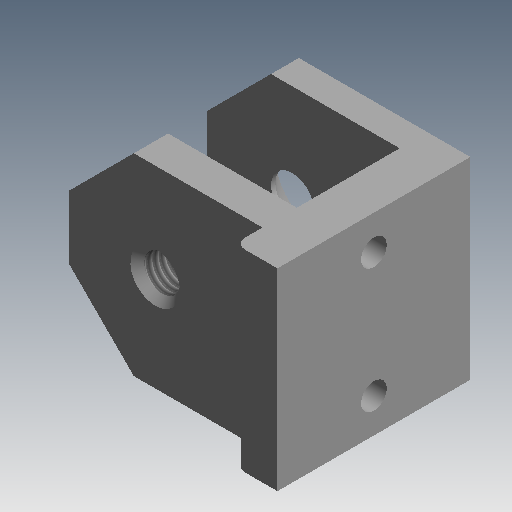
# Autodesk Inventor part: HBLTBBN45-SET_b
Saved by Autodesk Inventor 2020 (Build 240168000, 168)
## iProperties
Part Number: HBLTBBN45-SET_b
Material: 一般
Catalog Web Link: www.cadenas.de
Description: HBLTBA, HBLTBBNb-Free Angle Brackets - 20, 30, 40, 45 Square
Vendor: MISUMI
Document SubType Name: Modeling
Designer: partserver
Manufacturer: MISUMI
Mass: 44.0756 g
Surface Area: 143.656 cm^2
Volume: 44.0756 cm^3
Density: 1 g/cm^3
Appearance: PSOLRGB-192-192-192
Category: PARTsolutions
Company: MISUMI
PSOL_IDENT_0: {$CADENAS_DATA\23d-libs\misumi\metric\38_al_extrusions_blackets\hbltba.prj},183 {VTYP=3D},{NB=HBLTBB
PSOL_IDENT_1: N45-SET_b},{LINA=HBLTBBN45-SET},{NN=HBLTBA, HBLTBBNb},{DATE=08.06.2021 08:27:27},{GEOMDATE=18.10.201
PSOL_IDENT_2: 8 04:54:00},{VERSION=},{LINEID=100},{WBVAR=ALT1},{WBNUMERIC=}  {NB=HBLTBBN45-SET_b},{LINA=HBLTBBN45-
PSOL_IDENT_3: SET},{KT=DUMMY},{PN=HBLTBBN45-SET},{TP=HBLTBBN},{NO=45},{TNS=HBLTBBN45},{MATMB=A6N01SS-T5(Aluminum)(
PSOL_IDENT_4: EN AC-51400_AlMgSiO,7-T5)},{MATAB=SCM435(4137 Alloy Steel)(1.7220_34CrMo4)},{STMB=Alumite},{STAB=Tri
PSOL_IDENT_5: valent Chromate},{CS=45 Square (HFS8-45)},{A=45},{MA=6},{MAN=6},{N=-},{NN=0.0},{T=10},{TT1=6.5},{TT2=
PSOL_IDENT_6: 8.0},{W=24.0},{H=35},{H1=55},{E=29},{EN=29.0},{F=8},{FN=8.0},{C=15},{CN=15},{M=10},{L=16},{MASS=116.
PSOL_IDENT_7: 0},{AHS=M10x16},{ALT1=-SET},{ALT1ATT= '' , 'w/o Applicable Bolt and Nut Set' , '-SET' , 'with SET (A
PSOL_IDENT_8: pplicable Bolt and Nut Set)'   },{UM=-},{ACB=CBM6-35},{ACBD=6},{ACBDM=6},{ACBNO=6},{ACBL=35},{ACBQ=2
PSOL_IDENT_9: },{ACN=HDJFSN8-45},{ACNO=8-45},{ACNQ=1},{MATN=1010 Steel (or Equivalent)},{X=4},{MD=11.0},{AS=20.0},
PSOL_IDENT_10: {ES=5.5},{HFSH=6.000},{CPBL=27.6}
NB: HBLTBBN45-SET_b
NN: HBLTBA, HBLTBBNb
NT: Free Angle Brackets - 20, 30, 40, 45 Square
NBSYN: $PN._b
LINA: HBLTBBN45-SET
CATALOG: Misumi
PN: HBLTBBN45-SET
TNS: HBLTBBN45
MATMB: A6N01SS-T5
MATAB: 4137 Alloy Steel
STMB: Clear Anodizing
STAB: Trivalent Chromate Plating
CS: 45 Square (HFS8-45)
A: 45
MA: 6
N: -
T: 10
TT1: 6.5
TT2: 8
W: 24
H: 35
H1: 55
E: 29
F: 8
C: 15
M: 10
MASS: 116
AHS: M10x16
ALT1: with SET (Applicable Bolt and Nut Set)
UM: -
ACB: CBM6-35
ACBQ: 2
ACN: HDJFSN8-45
ACNQ: 1
MATN: 1010 Steel (or Equivalent)
AS: 20
ES: 5.5
SUPPLIER: MISUMI
ARTICLENO: HBLTBBN45-SET_b
BOMINFO: HBLTBBN45-SET
CREATOR: CADENAS GmbH
Title: HBLTBBN45-SET
Author: Cadenas PARTsolutions
Comments: Free Angle Brackets - 20, 30, 40, 45 Square
Autodesk Inventor part; units mm, degrees
ref_plane "YZ Plane" through (0, 0, 0) normal (1, 0, 0) x (0, 1, 0)
ref_plane "XZ Plane" through (0, 0, 0) normal (0, 1, 0) x (-1, 0, 0)
ref_plane "XY Plane" through (0, 0, 0) normal (0, 0, 1) x (1, 0, 0)
sketch "Sketch_6" plane through (0, 0, 0) normal (0, 0, 1) x (1, 0, 0)
  line L0 (0, 45) -> (0, 0)
  line L1 (0, 0) -> (7.5, 0)
  arc A0 (7.5, 0) -> (10, 2.5) centre (7.5, 2.5) ccw
  line L2 (10, 2.5) -> (10, 6.5)
  line L3 (10, 6.5) -> (55, 6.5)
  line L4 (55, 6.5) -> (55, 14.5)
  line L5 (55, 14.5) -> (10, 14.5)
  line L6 (10, 14.5) -> (10, 38.5)
  line L7 (10, 38.5) -> (55, 38.5)
  line L8 (55, 38.5) -> (55, 45)
  line L9 (55, 45) -> (0, 45)
  constraints: 20 end point, 2 point on circle, 1 centre point
extrude "Extrusion1" add sketch "Sketch_6" along normal mid plane 45
sketch "Sketch_7" plane through (0, 0, 0) normal (0, 1, 0) x (-1, 0, 0)
  line L0 (-40, 22.5) -> (-110, 22.5)
  line L1 (-110, 22.5) -> (-110, -22.5)
  line L2 (-110, -22.5) -> (-40, -22.5)
  line L3 (-40, -22.5) -> (-55, -7.5)
  line L4 (-55, -7.5) -> (-55, 7.5)
  line L5 (-55, 7.5) -> (-40, 22.5)
  constraints: 12 end point
extrude "Extrusion2" cut sketch "Sketch_7" along normal blind 45
sketch "Sketch_8" plane through (35, 0, 0) normal (1, 0, 0) x (0, 0, -1)
  line L0 (0, 6.5) -> (0, 14.5)
  line L1 (0, 14.5) -> (5, 14.5)
  line L2 (5, 14.5) -> (4.188, 13.688)
  line L3 (4.188, 13.688) -> (4.188, 8.112)
  line L4 (4.188, 8.112) -> (5.8, 6.5)
  line L5 (5.8, 6.5) -> (0, 6.5)
  line L6 (0, 6.5) -> (0, 14.5)
  constraints: 14 end point
revolve "Revolution1" cut sketch "Sketch_8" angle 360 about axis through (35, 6.5, 0) along (0, -1, 0)
thread "Thread1" size "M10x1.5" class "6H" standard "ISO Metric profile" full length
sketch "Sketch4" plane through (0, 45, 22.5) normal (0, 1, 0) x (1, 0, 0)
  point P0 (35, 22.5)
hole "Hole1" at (35, 45, 0) direction (0, -1, 0) diameter 10 depth 6.5 countersink diameter 21 countersink angle 90
sketch "Sketch5" plane through (0, 0, 22.5) normal (-1, 0, 0) x (0, 0, 1)
  point P0 (-37, 22.5)
hole "Hole2" at (0, 22.5, -14.5) direction (1, 0, 0) diameter 6 depth 10
sketch "Sketch6" plane through (0, 0, 22.5) normal (-1, 0, 0) x (0, 0, 1)
  point P0 (-8, 22.5)
hole "Hole3" at (0, 22.5, 14.5) direction (1, 0, 0) diameter 6 depth 10
ref_plane "bracket_to_screw_XY" through (35, 45, 0) normal (0, 1, 0) x (1, 0, 0)
ref_plane "bracket_to_screw_YZ" through (35, 45, 0) normal (1, 0, 0) x (0, 0, -1)
ref_plane "bracket_to_screw_ZX" through (35, 45, 0) normal (0, 0, -1) x (0, 1, 0)
ref_plane "screw11_XY" through (10, 22.5, 14.5) normal (1, 0, 0) x (0, 0, -1)
ref_plane "screw11_YZ" through (10, 22.5, 14.5) normal (0, 0, -1) x (0, 1, 0)
ref_plane "screw11_ZX" through (10, 22.5, 14.5) normal (0, 1, 0) x (1, 0, 0)
ref_plane "screw12_XY" through (10, 22.5, -14.5) normal (1, 0, 0) x (0, 0, -1)
ref_plane "screw12_YZ" through (10, 22.5, -14.5) normal (0, 0, -1) x (0, 1, 0)
ref_plane "screw12_ZX" through (10, 22.5, -14.5) normal (0, 1, 0) x (1, 0, 0)
ref_plane "screw1_1_XY" through (-27.6, 22.5, 14.5) normal (-1, 0, 0) x (0, 0, -1)
ref_plane "screw1_1_YZ" through (-27.6, 22.5, 14.5) normal (0, 0, -1) x (0, -1, 0)
ref_plane "screw1_1_ZX" through (-27.6, 22.5, 14.5) normal (0, -1, 0) x (-1, 0, 0)
ref_plane "screw1_2_XY" through (-27.6, 22.5, -14.5) normal (-1, 0, 0) x (0, 0, -1)
ref_plane "screw1_2_YZ" through (-27.6, 22.5, -14.5) normal (0, 0, -1) x (0, -1, 0)
ref_plane "screw1_2_ZX" through (-27.6, 22.5, -14.5) normal (0, -1, 0) x (-1, 0, 0)
ref_plane "screw2_XY" through (10, 22.5, 0) normal (1, 0, 0) x (0, 0, -1)
ref_plane "screw2_YZ" through (10, 22.5, 0) normal (0, 0, -1) x (0, 1, 0)
ref_plane "screw2_ZX" through (10, 22.5, 0) normal (0, 1, 0) x (1, 0, 0)
ref_plane "screw22_XY" through (2.2, 22.5, 0) normal (1, 0, 0) x (0, 0, -1)
ref_plane "screw22_YZ" through (2.2, 22.5, 0) normal (0, 0, -1) x (0, 1, 0)
ref_plane "screw22_ZX" through (2.2, 22.5, 0) normal (0, 1, 0) x (1, 0, 0)
ref_plane "screw3_XY" through (0, 22.5, 14.5) normal (1, 0, 0) x (0, 0, -1)
ref_plane "screw3_YZ" through (0, 22.5, 14.5) normal (0, 0, -1) x (0, 1, 0)
ref_plane "screw3_ZX" through (0, 22.5, 14.5) normal (0, 1, 0) x (1, 0, 0)
ref_plane "screw3_1_XY" through (0, 22.5, -14.5) normal (1, 0, 0) x (0, 0, -1)
ref_plane "screw3_1_YZ" through (0, 22.5, -14.5) normal (0, 0, -1) x (0, 1, 0)
ref_plane "screw3_1_ZX" through (0, 22.5, -14.5) normal (0, 1, 0) x (1, 0, 0)
body "Solid1"
